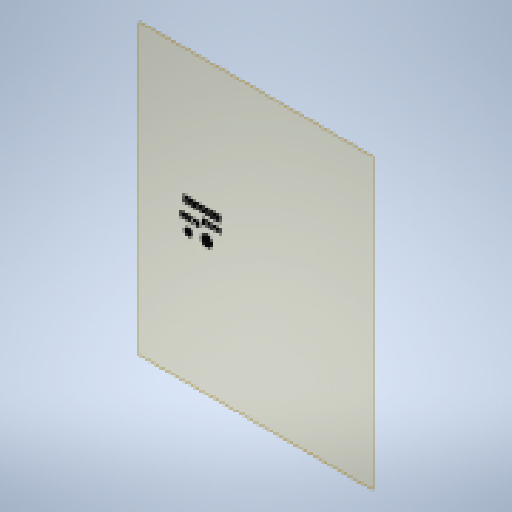
# Autodesk Inventor part: on-air-control-layout-2
Saved by Autodesk Inventor 2023 (Build 270158030, 158C)
## iProperties
Created: 2024-04-02
Part Number: on-air-control-layout-2
Material: Generic
Document SubType Name: Modeling
Designer: Imogen Heard
Density: 1 g/cm^3
Appearance: Default
Author: Imogen Heard
Autodesk Inventor part; units mm, degrees
ref_plane "YZ Plane" through (0, 0, 0) normal (1, 0, 0) x (0, 1, 0)
ref_plane "XZ Plane" through (0, 0, 0) normal (0, 1, 0) x (-1, 0, 0)
ref_plane "XY Plane" through (0, 0, 0) normal (0, 0, 1) x (1, 0, 0)
ref_plane "Work Plane1" through (0, 0, 0) normal (0, 0, 1) x (1, 0, 0)
sketch "Sketch1" plane through (0, 0, 0) normal (0, 0, 1) x (1, 0, 0)
  line L0 (-136.1347, 31.7782) -> (-66.1347, 31.7782)
  line L1 (-66.1347, 31.7782) -> (-66.1347, 19.7782)
  line L2 (-66.1347, 19.7782) -> (-136.1347, 19.7782)
  line L3 (-136.1347, 19.7782) -> (-136.1347, 31.7782)
  circle A0 centre (-126.1347, -24.2218) radius 8
  circle A1 centre (-126.1347, -24.2218) radius 10 construction
  circle A2 centre (-91.1347, -21.7218) radius 11
  circle A3 centre (-91.1347, -21.7218) radius 14.5 construction
  line L4 (-140.1347, 3.2782) -> (-105.1347, 3.2782)
  line L5 (-105.1347, 3.2782) -> (-105.1347, -6.7218)
  line L6 (-105.1347, -6.7218) -> (-140.1347, -6.7218)
  line L7 (-140.1347, -6.7218) -> (-140.1347, 3.2782)
  line L8 (-100.1347, 11.7782) -> (-65.1347, 11.7782)
  line L9 (-65.1347, 11.7782) -> (-65.1347, 1.7782)
  line L10 (-65.1347, 1.7782) -> (-100.1347, 1.7782)
  line L11 (-100.1347, 1.7782) -> (-100.1347, 11.7782)
  point P0 (0, 0)
  dimension "d0" = 70
  dimension "d1" = 12
  dimension "d2" = 16
  dimension "d3" = 20
  dimension "d4" = 22
  dimension "d5" = 29
  dimension "d6" = 10
  dimension "d7" = 35
  dimension "d8" = 10
  dimension "d9" = 35
  dimension "d11" = 8.5
  dimension "d12" = 25
  dimension "d13" = 2.5
  dimension "d14" = 35
  dimension "d15" = 5
  dimension "d16" = 20
  dimension "d17" = 15
  dimension "d77" = 14
  constraints: 24 end point, 6 parallel, 4 centre point, 3 horizontal, 3 perpendicular, 1 coincident
  measures "d0" distance between parallel lines of L1 L3
  measures "d1" distance between parallel lines of L2 L0
  measures "d2" diameter of A0
  measures "d3" diameter of A1
  measures "d4" diameter of A2
  measures "d5" diameter of A3
  measures "d6" distance between parallel lines of L6 L4
  measures "d7" distance between parallel lines of L7 L5
  measures "d8" distance between parallel lines of L10 L8
  measures "d9" distance between parallel lines of L11 L9
  measures "d11" distance between parallel lines of L4 L8
  measures "d12" distance from line of L1 A2.centre
  measures "d13" vertical distance of A0.centre A2.centre
  measures "d14" horizontal distance of A2.centre A0.centre
  measures "d15" distance between parallel lines of L11 L5
  measures "d16" distance between parallel lines of L8 L0
  measures "d17" distance from line of A2.centre L6
  measures "d77" distance from line of L5 A2.centre
extrude "Extrusion1" add sketch "Sketch1" along normal blind 1
sketch "Sketch2" plane through (0, 0, 1) normal (0, 0, 1) x (1, 0, 0)
  line L0 (-133.5304, 28.7782) -> (-67.3347, 28.7782) construction
  line L1 (-67.3347, 28.7782) -> (-67.3347, 21.7782) construction
  line L2 (-67.3347, 21.7782) -> (-133.5304, 21.7782) construction
  line L3 (-133.5304, 21.7782) -> (-133.5304, 28.7782) construction
  line L4 (-66.1347, 31.7782) -> (-136.1347, 31.7782) projected
  line L5 (-136.1347, 19.7782) -> (-66.1347, 19.7782) projected
  line L6 (-66.1347, 19.7782) -> (-66.1347, 31.7782) projected
  point P0 (0, 0)
  dimension "d82" = 3
  dimension "d83" = 2
  dimension "d84" = 1.2
  constraints: 1 horizontal alignment, 2 other
  measures "d82" distance between parallel lines of L4 L0
  measures "d83" distance between parallel lines of L5 L2
  measures "d84" distance between parallel lines of L6 L1
decal "Decal1"
sketch "Sketch3" plane through (0, 0, 1) normal (0, 0, 1) x (1, 0, 0)
  line L0 (-93.1347, 9.7782) -> (-67.5514, 9.7782) construction
  line L1 (-67.5514, 9.7782) -> (-67.5514, 3.7782) construction
  line L2 (-67.5514, 3.7782) -> (-93.1347, 3.7782) construction
  line L3 (-93.1347, 3.7782) -> (-93.1347, 9.7782) construction
  line L4 (-100.1347, 11.7782) -> (-100.1347, 1.7782) projected
  line L5 (-65.1347, 11.7782) -> (-100.1347, 11.7782) projected
  line L6 (-100.1347, 1.7782) -> (-65.1347, 1.7782) projected
  line L7 (-65.1347, 1.7782) -> (-65.1347, 11.7782) projected
  point P0 (0, 0)
  dimension "d85" = 7
  dimension "d88" = 2
  dimension "d91" = 2
  dimension "d92" = 6
  dimension "d93" = 2.4167
  constraints: 1 horizontal, 2 other
  measures "d85" distance between parallel lines of L4 L3
  measures "d88" distance between parallel lines of L5 L0
  measures "d91" distance between parallel lines of L6 L2
  measures "d92" distance of L0.end L1.end
  measures "d93" distance between parallel lines of L7 L1
decal "Decal2"
sketch "Sketch4" plane through (0, 0, 1) normal (0, 0, 1) x (1, 0, 0)
  line L0 (-135.6347, 1.2782) -> (-110.0514, 1.2782) construction
  line L1 (-110.0514, 1.2782) -> (-110.0514, -4.7218) construction
  line L2 (-110.0514, -4.7218) -> (-135.6347, -4.7218) construction
  line L3 (-135.6347, -4.7218) -> (-135.6347, 1.2782) construction
  line L4 (-140.1347, 3.2782) -> (-140.1347, -6.7218) projected
  line L5 (-105.1347, 3.2782) -> (-140.1347, 3.2782) projected
  line L6 (-140.1347, -6.7218) -> (-105.1347, -6.7218) projected
  line L7 (-105.1347, -6.7218) -> (-105.1347, 3.2782) projected
  point P0 (0, 0)
  dimension "d95" = 4.5
  dimension "d96" = 2
  dimension "d97" = 2
  dimension "d98" = 4.9167
  constraints: 2 other
  measures "d95" distance between parallel lines of L4 L3
  measures "d96" distance between parallel lines of L5 L0
  measures "d97" distance between parallel lines of L6 L2
  measures "d98" distance between parallel lines of L7 L1
decal "Decal3"
body "Solid1"
